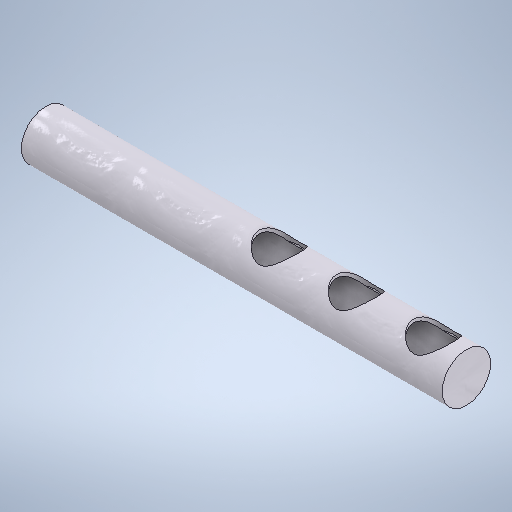
# Autodesk Inventor part: 102 part 2
Saved by Autodesk Inventor 2025.1 (Build 291241000, 241)
## iProperties
Created: 2024-07-24
Part Number: 102 part 2
Material: Aluminum 6061, geschweißt
Document SubType Name: Modeling
Designer: ffogue
Density: 2.7 g/cm^3
Appearance: Schweißnaht - Aluminum
Author: ffogue
Autodesk Inventor part; units mm, degrees
ref_plane "YZ Plane" through (0, 0, 0) normal (1, 0, 0) x (0, 1, 0)
ref_plane "XZ Plane" through (0, 0, 0) normal (0, 1, 0) x (-1, 0, 0)
sketch "Skizze1" plane through (0, 0, 0) normal (1, 0, 0) x (0, 1, 0)
  circle A0 centre (0, 0) radius 11
  dimension "d0" = 22
  constraints: 1 centre point, 1 coincident
  measures "d0" diameter of A0
extrude "Extrusion1" add sketch "Skizze1" along normal blind 191
shell "Wandung1" thickness 1.5 removed faces 1 at (0, -3.2467, -1.704)
ref_plane "Arbeitsebene1" through (0, 0, 11) normal (0, 0, 1) x (1, 0, 0)
sketch "Skizze2" plane through (0, 0, 11) normal (0, 0, 1) x (1, 0, 0)
  circle A0 centre (106, 0) radius 9
  circle A1 centre (141, 0) radius 9
  circle A2 centre (176, 0) radius 9
  line L0 (191, -11) -> (191, 11) projected
  line L1 (0, -11) -> (0, 11) projected
  point P0 (0, 0)
  dimension "d6" = 15
  dimension "d7" = 35
  dimension "d8" = 35
  dimension "d9" = 18
  constraints: 3 centre point, 3 horizontal alignment, 2 equal radius
  measures "d6" distance from line of L0 A2.centre
  measures "d7" distance of A2.centre A1.centre
  measures "d8" distance of A1.centre A0.centre
  measures "d9" diameter of A2
extrude "Extrusion2" cut sketch "Skizze2" against normal blind 6
